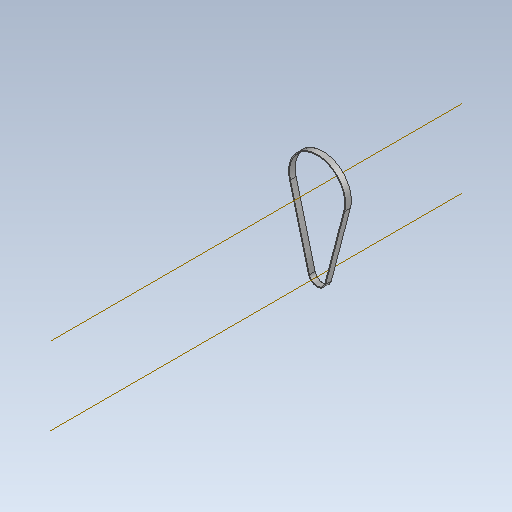
# Autodesk Inventor part: 0008-10-1015 Synchronous Belt2
Saved by Autodesk Inventor 2020 (Build 240168000, 168)
## iProperties
CustomPartVersion: 1
Created: 2020-05-28
Part Number: 0008-10-1015 Synchronous Belt2
Material: Rubber
Document SubType Name: Modeling
Designer: 40743
Density: 0.93 g/cm^3
Appearance: Rubber - Black - Version 1.1
Description: Curea Inchisa GT 2
Mass: 0.434783 g
Surface Area: 17.9212 cm^2
Volume: 0.467509 cm^3
Author: 40743
Subject: 1015
Autodesk Inventor part; units mm, degrees
sketch "Sketch Path" plane through (0, 0, 0) normal (0, 0, 1) x (1, 0, 0)
  arc A0 (1.7262, -1.5112) -> (13.2738, -1.5112) centre (7.5, 0) ccw
  arc A1 (26.7461, 49.9627) -> (-11.7461, 49.9627) centre (7.5, 55) ccw
  line L0 (26.7461, 49.9627) -> (13.2738, -1.5112)
  line L1 (1.7262, -1.5112) -> (-11.7461, 49.9627)
  constraints: 4 end point, 4 point on circle, 2 centre point
ref_plane "Cross Section Plane" through (13.2738, -1.5112, 0) normal (0.2532, 0.9674, 0) x (0, 0, 1)
ref_plane "Work Plane2" through (7.5, 0, 0) normal (-1, 0, 0) x (0, 0, 1)
ref_plane "Work Plane3" through (7.5, 55, 0) normal (0.2437, -0.9698, 0) x (0, 0, 1)
sketch "Cross Section" plane through (13.2738, -1.5112, 0) normal (0.2532, 0.9674, 0) x (0, 0, 1)
  line L0 (-2, 0.3) -> (2, 0.3)
  line L1 (2, 0.3) -> (2, -0.3)
  line L2 (2, -0.3) -> (-2, -0.3)
  line L3 (-2, -0.3) -> (-2, 0.3)
  line L4 (-2, 0) -> (2, 0) construction
  point P0 (0, 0)
  point P1 (0, 0)
  dimension "d0" = 4
  dimension "d4" = 0.3
  dimension "d5" = 0.3
  constraints: 10 end point, 3 midpoint, 2 parallel, 1 coincident, 1 horizontal, 1 perpendicular, 1 other
  measures "d0" distance between parallel lines of L1 L3
  measures "d4" distance between parallel lines of L2 L4
  measures "d5" distance between parallel lines of L4 L0
sweep "Belt" add profiles "Cross Section" path "Sketch Path"
equation "\"d0\" = da_B"
equation "\"d4\" = da_a"
equation "\"d5\" = da_a2"
equation "\"da_B\" = 4"
equation "\"da_pb\" = 2.5"
equation "\"da_L\" = 194.7953"
equation "\"da_a\" = 0.3"
equation "\"da_S\" = 1.5"
equation "\"da_Beta\" = 20deg"
equation "\"da_Ht\" = 0.7"
equation "\"da_H\" = 1.3"
equation "\"da_a2\" = 0.3"
body "Solid1"
